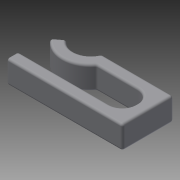
# Autodesk Inventor part: pinza
Saved by Autodesk Inventor 2015 SP1 (Build 190203100, 203)
## iProperties
Created: 2015-12-16
Part Number: pinza
Material: Generic
Document SubType Name: Modeling
Designer: pc
Density: 1 g/cm^3
Appearance: Default
Author: pc
Autodesk Inventor part; units mm, degrees
ref_plane "YZ Plane" through (0, 0, 0) normal (1, 0, 0) x (0, 1, 0)
ref_plane "XZ Plane" through (0, 0, 0) normal (0, 1, 0) x (-1, 0, 0)
ref_plane "XY Plane" through (0, 0, 0) normal (0, 0, 1) x (1, 0, 0)
sketch "Sketch1" plane through (0, 0, 0) normal (0, 0, 1) x (1, 0, 0)
  line L0 (-13.4572, -6) -> (9.0428, -6)
  line L1 (9.0428, -6) -> (9.0428, 0)
  line L2 (9.0428, 0) -> (-2.5, 0)
  arc A0 (-12.5, 0) -> (-2.5, 0) centre (-7.5, 3.75) ccw
  arc A1 (-10.5, 1.5) -> (-3.9645, 2.5) centre (-7.5, 3.75) ccw
  line L3 (-3.9645, 2.5) -> (11.5428, 2.5)
  line L4 (11.5428, 2.5) -> (11.5428, -8.5)
  line L5 (11.5428, -8.5) -> (-13.4572, -8.5)
  line L6 (-13.4572, -6) -> (-13.4572, -8.5)
  line L7 (-12.5, 0) -> (-10.5, 1.5)
  point P0 (0, 0)
  dimension "d4" = 6
  dimension "d5" = 25
  constraints: 16 end point, 4 point on circle, 2 centre point, 2 perpendicular, 1 horizontal, 1 vertical, 3 other
  measures "d4" distance of L0.end L1.end
  measures "d5" distance of L4.end L5.end
extrude "Extrusion1" add sketch "Sketch1" along normal blind 5
fillet "Fillet1" radius 2.8 2 edges at (9.0428, -6, 2.5) (9.0428, 0, 2.5)
fillet "Fillet2" radius 0.5 28 edges at (-3.6072, -6, 0) (-13.4572, -6, 2.5) (-3.6072, -6, 5) (1.8714, 0, 5) (-2.5, 0, 2.5) (1.8714, 0, 0) (-7.5, -2.5, 0) (-7.5, -2.5, 5) (-12.5, 0, 2.5) (-11.5, 0.75, 0) (-11.5, 0.75, 5) (-10.5, 1.5, 2.5) (-6.9328, 0.0431, 0) (-6.9328, 0.0431, 5) (-3.9645, 2.5, 2.5) (3.7892, 2.5, 0) (3.7892, 2.5, 5) (11.5428, 2.5, 2.5) (11.5428, -3, 0) (11.5428, -3, 5) (11.5428, -8.5, 2.5) (-0.9572, -8.5, 0) (-0.9572, -8.5, 5) (-13.4572, -8.5, 2.5) (-13.4572, -7.25, 0) (-13.4572, -7.25, 5) (8.2227, -5.1799, 0) (8.2227, -5.1799, 5)
body "Solid1"
